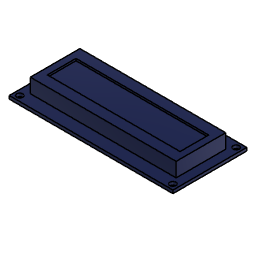
16x2 I2C LCD (Autodesk Fusion 360 design; units mm, degrees)
Autodesk Fusion 360 part; units mm, degrees
sketch "Sketch1" plane through (0, 0, 0) normal (0, 0, 1) x (1, 0, 0)
  line L0 (0, -20) -> (80.18, -20)
  line L1 (80.18, -20) -> (80.18, -56.15)
  line L2 (80.18, -56.15) -> (0, -56.15)
  line L3 (0, -56.15) -> (0, -20)
  line L4 (4.39, -25.94) -> (75.79, -25.94)
  line L5 (75.79, -25.94) -> (75.79, -50.21)
  line L6 (75.79, -50.21) -> (4.39, -50.21)
  line L7 (4.39, -50.21) -> (4.39, -25.94)
  line L8 (0, -20) -> (49, -20)
  line L9 (49, -20) -> (49, -40)
  line L10 (49, -40) -> (0, -40)
  line L11 (0, -40) -> (0, -20)
  line L12 (75.79, -38.075) -> (80.18, -38.075) construction
  line L13 (40.09, -25.94) -> (40.09, -20) construction
  line L14 (7.59, -31.075) -> (72.59, -31.075)
  line L15 (72.59, -31.075) -> (72.59, -45.075)
  line L16 (72.59, -45.075) -> (7.59, -45.075)
  line L17 (7.59, -45.075) -> (7.59, -31.075)
  line L18 (7.59, -38.075) -> (4.39, -38.075) construction
  line L19 (40.09, -31.075) -> (40.09, -25.94) construction
  circle A0 centre (2.59, -22.575) radius 1.5
  line L20 (2.59, -24.075) -> (7, -24.075) construction
  line L21 (4.09, -22.575) -> (4.09, -25) construction
  circle A1 centre (77.59, -22.575) radius 1.5
  line L22 (77.59, -24.075) -> (73.18, -24.075) construction
  line L23 (76.09, -22.575) -> (76.09, -25) construction
  circle A2 centre (77.59, -53.575) radius 1.5
  line L24 (76.09, -53.575) -> (76.09, -51.15) construction
  line L25 (77.59, -52.075) -> (73.18, -52.075) construction
  line L26 (2.59, -52.075) -> (7, -52.075) construction
  line L27 (4.09, -53.575) -> (4.09, -51.15) construction
  circle A3 centre (2.59, -53.575) radius 1.5
  line L28 (4.39, -25.94) -> (4.39, -20)
  line L29 (4.39, -25.94) -> (0, -25.94)
  line L30 (4.39, -34.7) -> (0, -34.7)
  line L31 (0, -34.7) -> (0, -40)
  line L32 (0, -40) -> (4.39, -40)
  line L33 (4.39, -40) -> (4.39, -34.7)
  dimension "d1020" = 20
  dimension "d1021" = 80.18
  dimension "d1022" = 36.15
  dimension "d1023" = 24.27
  dimension "d1024" = 71.4
  dimension "d1025" = 20
  dimension "d1026" = 49
  dimension "d1027" = 65
  dimension "d1028" = 14
  dimension "d1039" = 3
  dimension "d1040" = 28
  dimension "d1041" = 72
  dimension "d1212" = 14.7
  constraint horizontal L0
  constraint vertical L1
  constraint horizontal L2
  constraint vertical L3
  constraint horizontal L4
  constraint vertical L5
  constraint horizontal L6
  constraint vertical L7
  constraint horizontal L8
  constraint vertical L9
  constraint horizontal L10
  constraint vertical L11
  constraint midpoint L5 L12.start
  constraint midpoint L1 L12.end
  constraint midpoint L4 L13.start
  constraint midpoint L0 L13.end
  constraint vertical L13
  constraint horizontal L12
  constraint vertical origin L0.start
  constraint horizontal L14
  constraint vertical L15
  constraint horizontal L16
  constraint vertical L17
  constraint midpoint L17 L18.start
  constraint midpoint L7 L18.end
  constraint midpoint L14 L19.start
  constraint vertical L19
  constraint horizontal L18
  constraint coincident A0 L20.start
  constraint horizontal L20
  constraint coincident A0 L21.start
  constraint perpendicular L20 L21
  constraint tangent A0 L20
  constraint tangent A0 L21
  constraint symmetric L13 A0 A1
  constraint symmetric L13 L20.start L22.start
  constraint symmetric L13 L20.end L22.end
  constraint symmetric L13 L21.start L23.start
  constraint symmetric L13 L21.end L23.end
  constraint symmetric L18 A0 A3
  constraint symmetric L18 L20.start L26.start
  constraint symmetric L18 L20.end L26.end
  constraint symmetric L18 L21.start L27.start
  constraint symmetric L18 L21.end L27.end
  constraint symmetric L18 A1 A2
  constraint symmetric L18 L22.start L25.start
  constraint symmetric L18 L22.end L25.end
  constraint symmetric L18 L23.start L24.start
  constraint symmetric L18 L23.end L24.end
  constraint coincident L0 L28.end
  constraint coincident L11 L29.end
  constraint vertical L28
  constraint horizontal L29
  constraint horizontal L30
  constraint vertical L31
  constraint horizontal L32
  constraint vertical L33
  constraint collinear L7 L33
  measures "d1020" distance of origin L0.start
  measures "d1021" distance of L1 L3
  measures "d1022" distance of L0.start L2.end
  measures "d1023" distance of L4.end L5.end
  measures "d1024" distance of L5.end L6.end
  measures "d1025" distance of L8 L10
  measures "d1026" distance of L9.end L10.end
  measures "d1027" distance of L14.start L14.end
  measures "d1028" distance of L14.end L15.end
  measures "d1039" diameter of A0
  measures "d1040" distance of L20 L26
  measures "d1041" distance of L21 L23
  measures "d1212" distance of L8 L30
extrude "Extrude1" add sketch "Sketch1" against normal blind 1.53
extrude "Extrude2" add sketch "Sketch1" against normal blind 11 from surface at -1.53 contours L0 L4 L8 L9 L28 | L4 L7 L9 L10 L14 L17 L33 | L9 L10 L14 L17
extrude "Extrude3" add sketch "Sketch1" along normal blind 7 contours L4 L7 L9 L10 L14 L17 L33 | L4 L5 L6 L7 L9 L10 L14 L15 L16 L17 | L9 L10 L14 L15 L16 L17 | L9 L10 L14 L17
extrude "Extrude4" cut sketch "Sketch1" against normal blind 1 from surface at 7 contours L9 L10 L14 L15 L16 L17 | L9 L10 L14 L17
